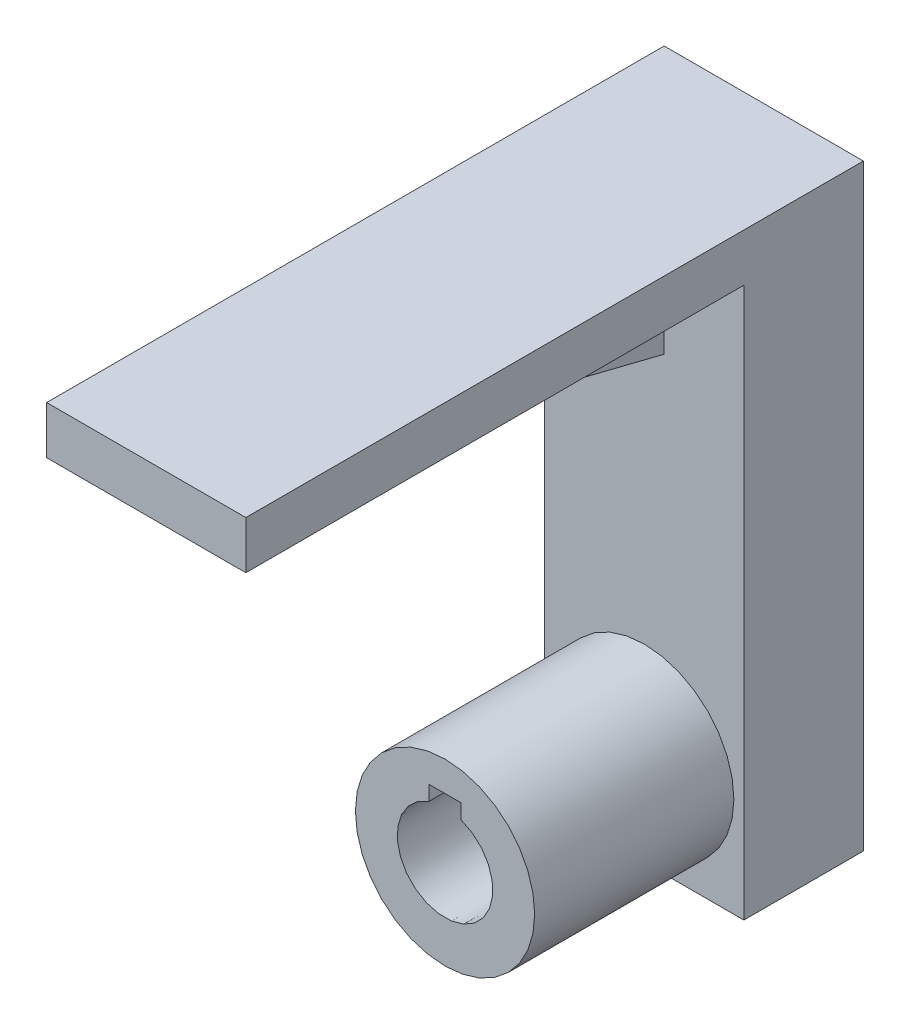
# Autodesk Inventor part: EndEffectorMotorAdapterOLD
Saved by Autodesk Inventor 2024 (Build 280153000, 153)
## iProperties
Created: 2024-02-13
Part Number: EndEffectorMotorAdapterOLD
Material: Generic
Document SubType Name: Modeling
Designer: yusuf
Density: 1 g/cm^3
Appearance: Default
Author: yusuf
Autodesk Inventor part; units mm, degrees
ref_plane "YZ Plane" through (0, 0, 0) normal (1, 0, 0) x (0, 1, 0)
ref_plane "XZ Plane" through (0, 0, 0) normal (0, 1, 0) x (-1, 0, 0)
ref_plane "XY Plane" through (0, 0, 0) normal (0, 0, 1) x (1, 0, 0)
sketch "Sketch7" plane through (0, 0, 0) normal (0, 0, 1) x (1, 0, 0)
  circle A0 centre (0, 0) radius 22.5
  dimension "d33" = 45
  constraints: 1 centre point, 1 coincident
  measures "d33" diameter of A0
extrude "Extrusion8" add sketch "Sketch7" along normal blind 50
sketch "Sketch8" plane through (0, 0, 50) normal (0, 0, 1) x (1, 0, 0)
  circle A0 centre (0, 0) radius 12
  line L0 (0, 0) -> (0, 15)
  line L1 (0, 15) -> (-4, 15)
  line L2 (-4, 15) -> (-4, 11.3137)
  line L3 (0, 15) -> (4, 15)
  line L4 (4, 15) -> (4, 11.3137)
  dimension "d36" = 24
  dimension "d37" = 15
  dimension "d38" = 4
  dimension "d39" = 4
  dimension "d40" = 3.6863
  constraints: 10 end point, 2 perpendicular, 2 point on circle, 2 vertical, 1 centre point, 1 coincident
  measures "d36" diameter of A0
  measures "d37" distance of L0.start L0.end
  measures "d38" distance of L0.end L1.end
  measures "d39" distance of L0.end L3.end
  measures "d40" distance of L3.end L4.end
extrude "Extrusion9" cut sketch "Sketch8" against normal blind 40
sketch "Sketch9" plane through (0, 0, 0) normal (0, 0, -1) x (-1, 0, 0)
  line L0 (-25, 25) -> (25, 25)
  line L1 (25, 25) -> (25, -25)
  line L2 (25, -25) -> (-25, -25)
  line L3 (-25, -25) -> (-25, 25)
  line L4 (-25, 25) -> (25, -25) construction
  line L5 (25, 25) -> (-25, -25) construction
  point P0 (0, 0)
  dimension "d43" = 50
  dimension "d44" = 50
  constraints: 12 end point, 2 midpoint, 2 parallel, 1 horizontal, 1 perpendicular
  measures "d43" distance of L0.end L1.end
  measures "d44" distance of L1.end L2.end
extrude "Extrusion10" add sketch "Sketch9" along normal blind 30
sketch "Sketch10" plane through (-25, 25, 0) normal (0, 1, 0) x (1, 0, 0)
  line L0 (50, 0) -> (0, 0) projected
  line L1 (50, 0) -> (50, 30) projected
  line L2 (0, 0) -> (50, 0)
  line L3 (50, 0) -> (50, 30)
  line L4 (50, 30) -> (0, 30)
  line L5 (0, 30) -> (0, 0)
  point P0 (25, 0)
  constraints: 8 end point, 2 parallel, 1 horizontal, 1 perpendicular
extrude "Extrusion11" add sketch "Sketch10" along normal blind 100
sketch "Sketch11" plane through (0, 0, 0) normal (0, 0, 1) x (1, 0, 0)
  line L0 (-25, -25) -> (-25, 125) projected
  line L1 (25, -25) -> (25, 125) projected
  line L2 (-25, 125) -> (25, 125)
  line L3 (25, 125) -> (25, 113)
  line L4 (25, 113) -> (-25, 113)
  line L5 (-25, 113) -> (-25, 125)
  point P0 (0, 0)
  dimension "d49" = 12
  constraints: 8 end point, 2 parallel, 1 horizontal, 1 perpendicular, 1 point on line
  measures "d49" distance between parallel lines of L2 L4
extrude "Extrusion12" add sketch "Sketch11" along normal blind 125
sketch "Sketch14" plane through (0, 0, 0) normal (1, 0, 0) x (0, 1, 0)
  line L0 (-25, 0) -> (113, 0) projected
  line L1 (113, 0) -> (88, 0)
  line L2 (-25, 0) -> (113, 0) projected
  line L3 (88, 0) -> (113, 100)
  point P0 (0, 0)
  dimension "d70" = 25
  dimension "d71" = 104.036
  dimension "d72" = 100
  constraints: 4 end point, 1 point on line
  measures "d70" distance of L0.end L1.end
  measures "d71" angle of L0 L3
  measures "d72" distance from line of L3.end L2
extrude "Rib2" add sketch "Sketch14" along normal mid plane 10 rib yes fills toward (100.5, 0.05) open curves L1 L3
body "Solid2"
